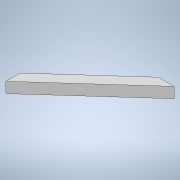
# Autodesk Inventor part: InnerDiagonalSupport
Saved by Autodesk Inventor 2020.1 (Build 241239000, 239)
## iProperties
Created: 2020-02-04
Part Number: InnerDiagonalSupport
Material: Generic
Document SubType Name: Modeling
Designer: super
Density: 1 g/cm^3
Appearance: Default
Author: super
Autodesk Inventor part; units mm, degrees
ref_plane "YZ Plane" through (0, 0, 0) normal (1, 0, 0) x (0, 1, 0)
ref_plane "XZ Plane" through (0, 0, 0) normal (0, 1, 0) x (-1, 0, 0)
ref_plane "XY Plane" through (0, 0, 0) normal (0, 0, 1) x (1, 0, 0)
sketch "Sketch1" plane through (0, 0, 0) normal (0, 1, 0) x (-1, 0, 0)
  line L0 (0, 0) -> (52.7633, 47.5083)
  line L1 (0, 0) -> (71, 0) construction
  line L2 (52.7633, 47.5083) -> (52.7633, 56.053)
  line L3 (52.7633, 56.053) -> (0, 8.5448)
  line L4 (0, 8.5448) -> (0, 0)
  dimension "d0" = 71
  dimension "d1" = 42
  constraints: 10 end point, 1 equal length, 1 horizontal, 1 parallel, 1 vertical
  measures "d0" distance of L0.start L0.end
  measures "d1" angle of L1 L0
extrude "Extrusion1" add sketch "Sketch1" along normal blind 6.35
sketch "Sketch2" plane through (0, 6.35, 0) normal (0, 1, 0) x (1, 0, 0)
  line L0 (-52.7633, -56.053) -> (0, -8.5448) projected
  line L1 (0, -8.5448) -> (-9.4899, -8.5448)
  line L2 (0, 0) -> (-52.7633, -47.5083) projected
  line L3 (0, -8.5448) -> (0, 0) projected
  line L4 (0, -8.5448) -> (0, 0)
  line L5 (0, 0) -> (-9.4899, -8.5448)
  constraints: 6 end point, 1 horizontal, 1 point on line, 1 vertical
extrude "Extrusion2" cut sketch "Sketch2" against normal blind 10
body "Solid1"
